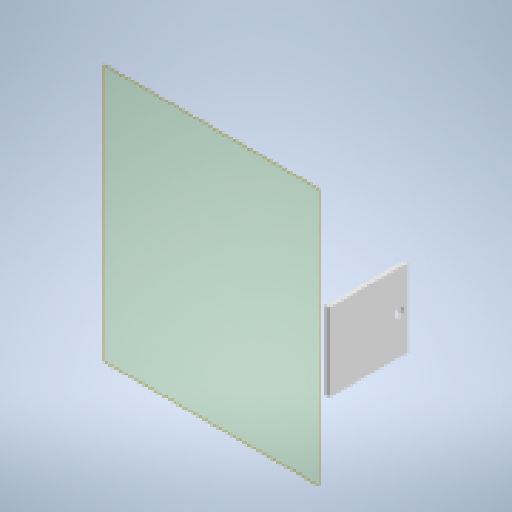
# Autodesk Inventor part: piano z
Saved by Autodesk Inventor 2024 (Build 280153000, 153)
## iProperties
Created: 2023-12-23
Part Number: piano z
Material: Generico
Document SubType Name: Modeling
Designer: Giorgio
Density: 1 g/cm^3
Appearance: Default
Author: Giorgio
Autodesk Inventor part; units mm, degrees
ref_plane "YZ Plane" through (0, 0, 0) normal (1, 0, 0) x (0, 1, 0)
ref_plane "XZ Plane" through (0, 0, 0) normal (0, 1, 0) x (-1, 0, 0)
ref_plane "XY Plane" through (0, 0, 0) normal (0, 0, 1) x (1, 0, 0)
ref_plane "Piano di lavoro1" through (-9.854, -197.5144, 1.4226) normal (0, 0, -1) x (1, 0, 0)
sketch "Schizzo1" plane through (-9.854, -197.5144, 1.4226) normal (0, 0, -1) x (1, 0, 0)
  line L0 (302.439, 120.7317) -> (292.439, 120.7317)
  line L1 (292.439, 120.7317) -> (292.439, -79.2683)
  line L2 (292.439, -79.2683) -> (302.439, -79.2683)
  line L3 (302.439, -79.2683) -> (302.439, 120.7317)
  point P0 (9.854, -197.5144)
  dimension "d0" = 200
  dimension "d1" = 10
  constraints: 8 end point, 2 parallel, 1 horizontal, 1 perpendicular
  measures "d0" distance of L2.end L0.start
  measures "d1" distance of L0.start L0.end
extrude "Estrusione1" add sketch "Schizzo1" along normal blind 200
sketch "Schizzo2" plane through (292.585, -318.2462, 1.4226) normal (1, 0, 0) x (0, 0, -1)
  circle A0 centre (180, 100) radius 11
  line L0 (0, 0) -> (200, 0)
  line L1 (200, 0) -> (200, 200)
  line L2 (200, 200) -> (0, 200)
  line L3 (0, 200) -> (0, 0)
  circle A1 centre (164.5, 84.5) radius 1.75
  circle A2 centre (164.5, 115.5) radius 1.75
  circle A3 centre (195.5, 115.5) radius 1.75
  circle A4 centre (195.5, 84.5) radius 1.75
  point P0 (200, 100)
  dimension "d4" = 22
  dimension "d5" = 200
  dimension "d6" = 200
  dimension "d7" = 100
  dimension "d9" = 31
  dimension "d10" = 31
  dimension "d11" = 15.5
  dimension "d12" = 31
  dimension "d13" = 31
  dimension "d14" = 0
  dimension "d15" = 15.5
  dimension "d16" = 0
  dimension "d17" = 3.5
  dimension "d18" = 3.5
  dimension "d19" = 3.5
  dimension "d20" = 3.5
  dimension "d22" = 20
  constraints: 8 end point, 5 centre point, 2 parallel, 1 horizontal, 1 midpoint, 1 perpendicular
  measures "d4" diameter of A0
  measures "d5" distance of L2.end L1.end
  measures "d6" distance of L1.end L0.end
  measures "d7" distance from line of A0.centre L0
  measures "d9" distance of A4.centre A1.centre
  measures "d10" distance of A3.centre A2.centre
  measures "d11" horizontal distance of A0.centre A2.centre
  measures "d12" distance of A1.centre A2.centre
  measures "d13" distance of A4.centre A3.centre
  measures "d14" horizontal distance of A2.centre A1.centre
  measures "d15" horizontal distance of A0.centre A4.centre
  measures "d16" vertical distance of A4.centre A1.centre
  measures "d17" diameter of A1
  measures "d18" diameter of A2
  measures "d19" diameter of A3
  measures "d20" diameter of A4
  measures "d22" distance of point (200, 100) A0.centre
extrude "Estrusione2" cut sketch "Schizzo2" against normal blind 10 contours A0 | A1 | A2 | A3 | A4
equation "\"d10\" = d9"
equation "\"d11\" = 0.5 * d9"
equation "\"d12\" = d9"
equation "\"d13\" = d9"
equation "\"d15\" = 0.5 * d9"
equation "\"d18\" = d17"
equation "\"d19\" = d17"
equation "\"d20\" = d17"
